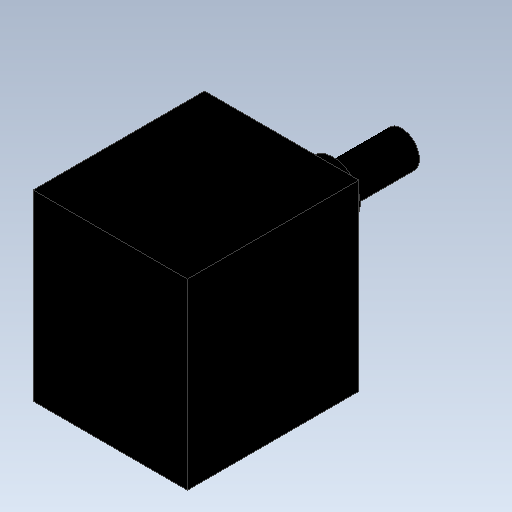
# Autodesk Inventor part: encoder
Saved by Autodesk Inventor 2020 (Build 240168000, 168)
## iProperties
Created: 2017-11-25
Part Number: encoder
Material: Generic
Document SubType Name: Modeling
Designer: stedrock
Density: 1 g/cm^3
Appearance: Default
Mass: 26.8943 g
Surface Area: 57.6574 cm^2
Volume: 26.8943 cm^3
Author: stedrock
Autodesk Inventor part; units mm, degrees
ref_plane "YZ Plane" through (0, 0, 0) normal (1, 0, 0) x (0, 1, 0)
ref_plane "XZ Plane" through (0, 0, 0) normal (0, 1, 0) x (-1, 0, 0)
ref_plane "XY Plane" through (0, 0, 0) normal (0, 0, 1) x (1, 0, 0)
sketch "Sketch1" plane through (0, 0, 0) normal (0, 0, 1) x (1, 0, 0)
  line L0 (-13.5, -16) -> (13.5, -16)
  line L1 (13.5, -16) -> (13.5, 16)
  line L2 (13.5, 16) -> (-13.5, 16)
  line L3 (-13.5, 16) -> (-13.5, -16)
  line L4 (-13.5, -16) -> (13.5, 16) construction
  line L5 (13.5, -16) -> (-13.5, 16) construction
  line L6 (0, 0) -> (0, 25.8288) construction
  circle A0 centre (0, 3.5) radius 4.75
  circle A1 centre (0, 3.5) radius 3.1
  line L7 (2.1901, 1.3061) -> (-2.1901, 1.3061)
  dimension "d0" = 27
  dimension "d1" = 32
  dimension "d4" = 9.5
  dimension "d5" = 12.5
  dimension "d8" = 6.2
  constraints: 16 end point, 2 centre point, 2 horizontal, 2 midpoint, 2 parallel, 2 point on circle, 1 coincident, 1 perpendicular, 1 point on line, 1 vertical
  measures "d0" distance of L2.end L1.end
  measures "d1" distance of L1.end L0.end
  measures "d4" diameter of A0
  measures "d5" distance from line of L2 A0.centre
  measures "d8" diameter of A1
extrude "Extrusion1" add sketch "Sketch1" along normal blind 30 contours L3 L2 L1 L0 | A0 | A1 L7 | L7 A1
extrude "Extrusion2" add sketch "Sketch1" against normal blind 9 contours A0 | A1 L7 | L7 A1
extrude "Extrusion3" add sketch "Sketch1" against normal blind 21 contours A1 L7 picked at (0.101, 3.0658)
extrude "Extrusion4" add sketch "Sketch1" against normal blind 11.5 contours A1 L7 | L7 A1
body "Solid1"
